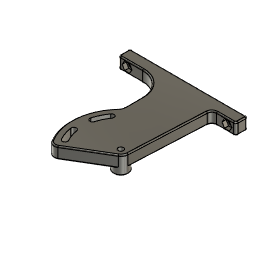
BalanceFrameFront v2 (Autodesk Fusion 360 design; units mm, degrees)
Autodesk Fusion 360 part; units mm, degrees
sketch "main" plane through (0, 0, 0) normal (0, 0, 1) x (1, 0, 0)
  line L0 (-42.914809, 50.281849) -> (54.085191, 50.281849)
  line L1 (55.585191, 48.781849) -> (55.585191, 42.281849)
  line L2 (-44.414809, 42.281849) -> (-44.414809, 48.781849)
  circle A0 centre (25.87268, -27.77406) radius 6.25
  line L3 (-3.06435, -52.399215) -> (29.085121, -33.135284)
  line L4 (35.193281, 36.472366) -> (32.115587, -28.071744)
  circle A1 centre (25.87268, -27.77406) radius 2.25
  line L5 (30.02768, -27.77406) -> (27.95018, -24.175724)
  line L6 (27.95018, -24.175724) -> (23.79518, -24.175724)
  line L7 (23.79518, -24.175724) -> (21.71768, -27.77406)
  line L8 (21.71768, -27.77406) -> (23.79518, -31.372395)
  line L9 (23.79518, -31.372395) -> (27.95018, -31.372395)
  line L10 (27.95018, -31.372395) -> (30.02768, -27.77406)
  arc A2 (-5.067004, 1.363304) -> (-9.835233, -50.821726) centre (25.87268, -27.77406) ccw
  arc A3 (-9.835233, -50.821726) -> (-3.06435, -52.399215) centre (-5.634302, -48.110236) ccw
  arc A4 (-9.948645, -17.556666) -> (-5.621237, -18.790982) centre (-7.784941, -18.173824) ccw
  arc A5 (-0.744437, -8.692875) -> (-4.40175, -6.071033) centre (-2.573093, -7.381954) ccw
  arc A6 (-6.460462, -32.982748) -> (-10.903184, -33.698445) centre (-8.681823, -33.340596) ccw
  arc A7 (-6.724824, -45.800851) -> (-2.786871, -43.623118) centre (-4.755848, -44.711984) ccw
  arc A8 (-4.40175, -6.071033) -> (-9.948645, -17.556666) centre (25.87268, -27.77406) ccw
  arc A9 (-10.903184, -33.698445) -> (-6.724824, -45.800851) centre (25.87268, -27.77406) ccw
  arc A10 (-0.744437, -8.692875) -> (-5.621237, -18.790982) centre (25.87268, -27.77406) ccw
  arc A11 (-6.460462, -32.982748) -> (-2.786871, -43.623118) centre (25.87268, -27.77406) ccw
  line L11 (-3.706967, 4.791229) -> (-3.706967, 20.281849)
  line L12 (53.585191, 40.281849) -> (39.188741, 40.281849)
  line L13 (-23.706967, 40.281849) -> (-42.414809, 40.281849)
  arc A12 (-3.706967, 20.281849) -> (-23.706967, 40.281849) centre (-23.706967, 20.281849) ccw
  arc A13 (39.188741, 40.281849) -> (35.193281, 36.472366) centre (39.188741, 36.281849) ccw
  arc A14 (53.585191, 40.281849) -> (55.585191, 42.281849) centre (53.585191, 42.281849) ccw
  arc A15 (-44.414809, 42.281849) -> (-42.414809, 40.281849) centre (-42.414809, 42.281849) ccw
  arc A16 (-42.914809, 50.281849) -> (-44.414809, 48.781849) centre (-42.914809, 48.781849) ccw
  arc A17 (55.585191, 48.781849) -> (54.085191, 50.281849) centre (54.085191, 48.781849) ccw
  arc A18 (-5.067004, 1.363304) -> (-3.706967, 4.791229) centre (-8.706967, 4.791229) ccw
  point P0 (-44.414809, 50.281849)
  point P1 (55.585191, 50.281849)
  point P2 (-44.414809, 40.281849)
  point P3 (25.87268, -27.77406)
  dimension "d1" = 100
  dimension "d2" = 10
  dimension "d3" = 92.73
  dimension "d4" = 123.66
  dimension "d5" = 12.5
  dimension "d6" = 4.5
  dimension "d7" = 4.155
  dimension "d8" = 85
  dimension "d9" = 5
  dimension "d10" = 65.5
  dimension "d11" = 4.5
  dimension "d13" = 4.5
  dimension "d14" = 4.5
  dimension "d15" = 4.5
  dimension "d16" = 20
  dimension "d17" = 4
  dimension "d18" = 2
  dimension "d19" = 1.5
  dimension "d20" = 5
  constraint horizontal L0
  constraint vertical L1
  constraint horizontal L12
  constraint vertical L2
  constraint tangent A0 L4
  constraint tangent A0 L3
  constraint concentric A0 A1
  constraint tangent A2 A3
  constraint tangent L3 A3
  constraint concentric A1 A10
  constraint tangent A5 A10
  constraint concentric A8 A10
  constraint tangent A4 A10
  constraint tangent A6 A10
  constraint tangent A7 A10
  constraint concentric A8 A9
  constraint concentric A10 A11
  constraint perpendicular L11 L12
  constraint collinear L12 L13
  constraint tangent L13 A12
  constraint tangent L11 A12
  constraint tangent L12 A13
  constraint tangent L4 A13
  constraint tangent L12 A14
  constraint tangent L1 A14
  constraint tangent L13 A15
  constraint tangent L2 A15
  constraint equal A14 A15
  constraint tangent L2 A16
  constraint tangent L0 A16
  constraint tangent L1 A17
  constraint tangent L0 A17
  constraint equal A16 A17
  constraint tangent A2 A18
  constraint tangent L11 A18
  measures "d3" angle of L4 L12
  measures "d4" angle of L3 L4
  measures "d5" diameter of A0
  measures "d6" diameter of A1
  measures "d8" diameter of A2
  measures "d9" radius of A3
  measures "d10" diameter of A10
  measures "d11" diameter of A5
  measures "d13" diameter of A4
  measures "d14" diameter of A6
  measures "d15" diameter of A7
  measures "d16" radius of A12
  measures "d17" radius of A13
  measures "d18" radius of A14
  measures "d19" radius of A16
  measures "d20" radius of A18
extrude "Extrude1" add sketch "main" along normal blind 10 contours L0 L1 L2 A0 L3 L4 A2 A3 L11 L12 L13 A12 A13 A14 A15 A16 A17 A18 picked at (19.048744, 6.578638)
extrude "Extrude2" add sketch "main" along normal blind 10 and the other way blind 5.5 contours A0 | L5 L6 L7 L8 L9 L10 picked at (21.982566, -25.547625) picked at (25.816633, -30.920853)
extrude "Extrude3" cut sketch "main" along normal blind -5.5 and the other way blind 1.5 contours L5 L6 L7 L8 L9 L10 picked at (25.816633, -30.920853)
sketch "holes" plane through (0, 40.281849, 0) normal (0, -1, 0) x (1, 0, 0)
  line L0 (-42.414809, 0) -> (-23.706967, 0)
  line L1 (-23.706967, 0) -> (-23.706967, 10)
  line L2 (-23.706967, 10) -> (-42.414809, 10)
  line L3 (-42.414809, 10) -> (-42.414809, 0)
  line L4 (-42.414809, 10) -> (-36.914809, 10)
  line L5 (-42.414809, 5) -> (-42.414809, 10)
  circle A0 centre (-36.914809, 5) radius 2.25
  line L6 (-41.069809, 5) -> (-38.992309, 1.401664)
  line L7 (-38.992309, 1.401664) -> (-34.837309, 1.401664)
  line L8 (-34.837309, 1.401664) -> (-32.759809, 5)
  line L9 (-32.759809, 5) -> (-34.837309, 8.598336)
  line L10 (-34.837309, 8.598336) -> (-38.992309, 8.598336)
  line L11 (-38.992309, 8.598336) -> (-41.069809, 5)
  line L12 (53.585191, 10) -> (48.085191, 10)
  line L13 (53.585191, 5) -> (53.585191, 10)
  circle A1 centre (48.085191, 5) radius 2.25
  line L14 (52.240191, 5) -> (50.162691, 8.598336)
  line L15 (50.162691, 8.598336) -> (46.007691, 8.598336)
  line L16 (46.007691, 8.598336) -> (43.930191, 5)
  line L17 (43.930191, 5) -> (46.007691, 1.401664)
  line L18 (46.007691, 1.401664) -> (50.162691, 1.401664)
  line L19 (50.162691, 1.401664) -> (52.240191, 5)
  point P0 (-36.914809, 5)
  point P1 (53.585191, 10)
  point P2 (48.085191, 5)
  dimension "d31" = 5.5
  dimension "d32" = 5
  dimension "d33" = 4.5
  dimension "d34" = 4.155
  dimension "d35" = 5.5
  dimension "d36" = 5
  dimension "d37" = 4.5
  dimension "d38" = 4.155
  constraint horizontal L4
  constraint vertical L5
  constraint horizontal L12
  constraint vertical L13
  measures "d33" diameter of A0
  measures "d37" diameter of A1
extrude "Extrude4" cut sketch "holes" against normal blind 20 contours A0 | A1 picked at (-36.11341, 5.586374) picked at (48.88659, 5.586374)
extrude "Extrude5" cut sketch "holes" against normal blind 3.5 contours L6 L7 L8 L9 L10 L11 | L14 L15 L16 L17 L18 L19 picked at (-34.161582, 6.524858) picked at (45.331965, 3.475142)
fillet "Fillet1" radius 1 36 edges at (33.654434, 4.200311, 0) (36.428494, 39.17685, 0) (46.386966, 40.281849, 0) (54.999405, 40.867635, 0) (55.585191, 45.531849, 0) (55.145851, 49.842509, 0) (5.585191, 50.281849, 0) (-43.975469, 49.842509, 0) (-44.414809, 45.531849, 0) (-43.829022, 40.867635, 0) (-33.060888, 40.281849, 0) (-9.564831, 34.423984, 0) (-3.706967, 12.536539, 0) (-4.059397, 2.947295, 0) (-16.451012, -23.906877, 0) (-6.768825, -52.979821, 0) (13.010385, -42.76725, 0) (33.654434, 4.200311, 10) (36.428494, 39.17685, 10) (46.386966, 40.281849, 10) (54.999405, 40.867635, 10) (55.585191, 45.531849, 10) (55.145851, 49.842509, 10) (5.585191, 50.281849, 10) (-43.975469, 49.842509, 10) (-44.414809, 45.531849, 10) (-43.829022, 40.867635, 10) (-33.060888, 40.281849, 10) (-9.564831, 34.423984, 10) (-3.706967, 12.536539, 10) (-4.059397, 2.947295, 10) (-16.451012, -23.906877, 10) (-6.768825, -52.979821, 10) (13.010385, -42.76725, 10) (31.235586, -30.983692, 10) (20.045634, -25.513963, -5.5)
equation "d7 = ( 8.31 / 2 ) * 1 mm"
equation "d34 = ( 8.31 / 2 ) * 1 mm"
equation "d38 = ( 8.31 / 2 ) * 1 mm"
